e48acfb7-4e08-4e2e-8d3e-d02aebe9fb48 (Autodesk Fusion 360 design; units mm, degrees)
Autodesk Fusion 360 part; units mm, degrees
sketch "Sketch2" plane through (0, 0, 0) normal (1, 0, 0) x (0, 1, 0)
  line L0 (0, 0) -> (12.7, 0) construction
  line L1 (25.7556, 0) -> (12.7, 0) construction
  circle A0 centre (19.2278, 0) radius 6.5278
  dimension "d1" = 12.7
  dimension "d2" = 25.7556
  constraint coincident L0.start origin
  constraint horizontal L0
  constraint parallel L0 L1
  constraint midpoint L1 A0.centre
  constraint coincident L1.start A0
  measures "d1" distance of L0.start L0.end
  measures "d2" distance of L0.start L1.start
revolve "Revolve4" add sketch "Sketch2" angle 360 about axis through (0, 0, 1.75) along (0, 0, 1) makes body 1
ref_plane "WorkPlane1" through (-25.7556, 0, 0) normal (1, 0, 0) x (0, 1, 0)
ref_plane "WorkPlane2" through (47.2694, 0, 0) normal (1, 0, 0) x (0, 1, 0)
ref_plane "WorkPlane3" through (28.2194, 0, 0) normal (1, 0, 0) x (0, 1, 0)
sketch "Sketch6" plane through (28.2194, 0, 0) normal (1, 0, 0) x (0, 1, 0)
  circle A0 centre (0, 0) radius 4.7625
  dimension "d31" = 9.525
  constraint coincident A0.centre origin
  measures "d31" diameter of A0
extrude "Extrude1" add sketch "Sketch6" along normal up to surface (19.05 mm away) separate body makes body 2
ref_plane "WorkPlane4" through (19.2278, 0, 0) normal (1, 0, 0) x (0, 1, 0)
sketch "Sketch7" plane through (0, 0, 0) normal (0, 0, 1) x (1, 0, 0)
  line L0 (19.2278, 0.75) -> (19.2278, 21.75)
  line L1 (0, 0) -> (76.2, 0) construction
  line L2 (19.2278, 18.7283) -> (19.2278, -25.4) construction
  line L3 (19.2278, 0) -> (33.5153, 0)
  line L4 (33.5153, 0) -> (33.5153, 8.4388)
  line L5 (19.2278, 0) -> (19.2278, 4.7625)
  line L6 (30.8047, 10.1651) -> (19.2278, 4.7625)
  arc A0 (33.5153, 8.4388) -> (30.8047, 10.1651) centre (31.6103, 8.4388) ccw
  point P0 (33.5153, 11.43)
  dimension "d40" = 14.2875
  dimension "d41" = 11.43
  dimension "d42" = 4.7625
  dimension "d43" = 1.905
  constraint coincident L1.start origin
  constraint horizontal L1
  constraint coincident L0 L2.start
  constraint parallel L0 L2
  constraint coincident L2 L3.start
  constraint coincident L1 L3.start
  constraint perpendicular L2 L3
  constraint perpendicular L3 L4
  constraint perpendicular L3 L5
  constraint coincident P0 L4
  constraint coincident P0 L6
  constraint tangent L4 A0
  constraint tangent L6 A0
  measures "d40" distance of L3.start L3.end
  measures "d41" distance of L3.end P0
  measures "d42" distance of L3.start L5.end
  measures "d43" radius of A0
revolve "Revolve5" add sketch "Sketch7" angle 360 about axis through (0, 0, 0) along (1, 0, 0) bodies 1 2
thread "Thread2" "ANSI Unified Screw Threads 0.3125 5/16-18 UNC 3A" major diameter 7.8283 minor diameter 6.2586 pitch 1.4111 angle 60 modelled right hand crest width 0.2172 on face at (38.1, 4.7388, 0.4742) crest through (33.1625, 3.9141, 0) on bodies 1
fillet "Fillet2" radius 1.905 1 edges at (24.6927, -7.3094, 0.2219) on bodies 1
equation "d27 = -d2"
equation "d28 = 2.875 in"
equation "d30 = -0.750 in"
equation "EyeInner = d1"
equation "EyeOuter = d2"
equation "ThreadDia = d31"
equation "TotalLength = d28"
equation "ShankLength = d30"
equation "d39 = d1 + ( ( d2 - d1 ) ) / 2"
equation "d40 = d31 * 1.5"
equation "d41 = d31 * 1.2"
equation "d42 = d31 / 2"
equation "d43 = d31 * 0.2"
equation "d45 = d31 * 0.2"
